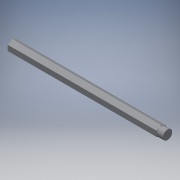
# Autodesk Inventor part: Hex Shaft
Saved by Autodesk Inventor 2018 (Build 220112000, 112)
## iProperties
Created: 2019-01-19
Part Number: Hex Shaft
Material: Generic
Document SubType Name: Modeling
Designer: Gabriel
Density: 1 g/cm^3
Appearance: Default
Author: Gabriel
Autodesk Inventor part; units mm, degrees
ref_plane "YZ Plane" through (0, 0, 0) normal (1, 0, 0) x (0, 1, 0)
ref_plane "XZ Plane" through (0, 0, 0) normal (0, 1, 0) x (-1, 0, 0)
ref_plane "XY Plane" through (0, 0, 0) normal (0, 0, 1) x (1, 0, 0)
sketch "Sketch1" plane through (0, 0, 0) normal (1, 0, 0) x (0, 1, 0)
  line L0 (0, 1.5838) -> (0, -3.1787)
  line L1 (-2.7424, -3.1787) -> (-5.4957, 1.5775)
  line L2 (-5.4957, 1.5775) -> (-2.7532, 6.34)
  line L3 (-2.7532, 6.34) -> (2.7424, 6.3463)
  line L4 (2.7424, 6.3463) -> (5.4957, 1.59)
  line L5 (5.4957, 1.59) -> (2.7532, -3.1725)
  line L6 (2.7532, -3.1725) -> (-2.7424, -3.1787)
  point P0 (0, 0)
  dimension "d0" = 4.7625
  constraints: 14 end point, 1 coincident, 1 vertical, 13 other
  measures "d0" distance of L0.start L0.end
extrude "Extrusion1" add sketch "Sketch1" along normal blind 152.4
sketch "Sketch2" plane through (152.4, 0, 0) normal (1, 0, 0) x (0, 0, -1)
  line L0 (3.1725, 2.7532) -> (-1.59, 5.4957) projected
  line L1 (0.7913, 4.1244) -> (-1.5775, -0.0072)
  circle A0 centre (-1.5775, -0.0072) radius 4.7625
  point P0 (0, 0)
  dimension "d3" = 4.7625
  constraints: 2 end point, 1 coincident, 1 midpoint, 3 other
  measures "d3" distance of L1.start L1.end
extrude "Extrusion2" add sketch "Sketch2" along normal blind 6.35
body "Solid1"
